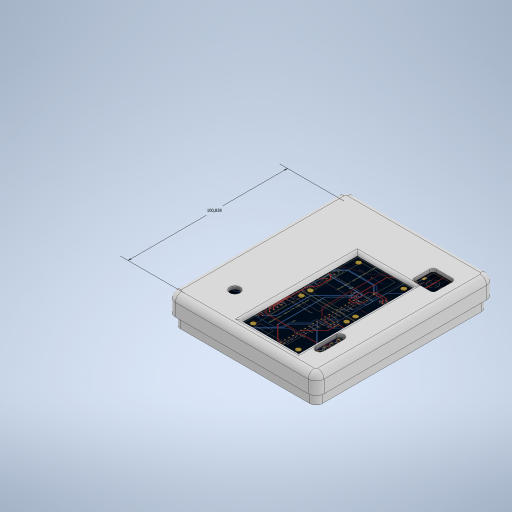
# Autodesk Inventor part: lid_lautering_tank
Saved by Autodesk Inventor 2024.4 (Build 284460000, 460)
## iProperties
Created: 2026-05-24
Part Number: lid_lautering_tank
Material: Generic
Document SubType Name: Modeling
Designer: Emil
Density: 1 g/cm^3
Appearance: Default
Author: Emil
Autodesk Inventor part; units mm, degrees
ref_plane "YZ Plane" through (0, 0, 0) normal (1, 0, 0) x (0, 1, 0)
ref_plane "XZ Plane" through (0, 0, 0) normal (0, 1, 0) x (-1, 0, 0)
ref_plane "XY Plane" through (0, 0, 0) normal (0, 0, 1) x (1, 0, 0)
sketch "Sketch1" plane through (0, 0, 0) normal (0, 1, 0) x (-1, 0, 0)
  line L0 (0, 0) -> (0, -100.838) construction
  line L1 (0, -100.838) -> (-82.0304, -100.838) construction
  line L2 (-82.0304, -100.838) -> (-82.0304, 0) construction
  line L3 (-82.0304, 0) -> (0, 0) construction
  dimension "d3" = 100.838
  constraints: 2 other
  measures "d3" distance of L0.start L0.end
sketch "Sketch2" plane through (0, 0, 0) normal (0, 1, 0) x (-1, 0, 0)
  line L0 (0, 0) -> (0, -100.838) construction
  line L1 (-82.0304, 0) -> (0, 0) construction
  line L2 (0, -100.838) -> (-82.0304, -100.838) construction
  line L3 (-82.0304, -100.838) -> (-82.0304, 0) construction
  line L4 (0, -50.419) -> (-82.0304, -50.419) construction
  line L5 (-41.0152, -50.419) -> (-41.0152, -100.838) construction
  line L6 (-41.0152, -50.419) -> (-41.0152, 0) construction
  line L7 (-85.8804, 3.85) -> (3.85, 3.85)
  line L8 (3.85, 3.85) -> (3.85, -104.688)
  line L9 (3.85, -104.688) -> (-85.8804, -104.688)
  line L10 (-85.8804, -104.688) -> (-85.8804, 3.85)
  line L11 (-85.8804, 3.85) -> (3.85, -104.688) construction
  line L12 (3.85, 3.85) -> (-85.8804, -104.688) construction
  line L13 (-88.0304, 6) -> (6, 6)
  line L14 (6, 6) -> (6, -106.838)
  line L15 (6, -106.838) -> (-88.0304, -106.838)
  line L16 (-88.0304, -106.838) -> (-88.0304, 6)
  line L17 (-88.0304, 6) -> (6, -106.838) construction
  line L18 (6, 6) -> (-88.0304, -106.838) construction
  dimension "d8" = 2.15
  dimension "d9" = 3.85
  dimension "d10" = 3.85
  dimension "d11" = 2.15
  dimension "d39" = 94.0304
  dimension "d40" = 112.838
  constraints: 30 end point, 9 midpoint, 4 parallel, 2 horizontal, 2 perpendicular, 1 other
  measures "d8" distance between parallel lines of L8 L14
  measures "d9" distance between parallel lines of L2 L9
  measures "d10" distance between parallel lines of L8 L0
  measures "d11" distance between parallel lines of L9 L15
  measures "d39" distance of L13.start L13.end
  measures "d40" distance of L15.end L13.start
extrude "Extrusion1" add sketch "Sketch2" against normal blind 10
sketch "Sketch3" plane through (0, 0, 0) normal (0, 1, 0) x (1, 0, 0)
  line L0 (88.0304, -6) -> (-6, -6) projected
  line L1 (-6, 106.838) -> (88.0304, 106.838) projected
  line L2 (-6, -6) -> (88.0304, -6)
  line L3 (88.0304, -6) -> (88.0304, 106.838)
  line L4 (88.0304, 106.838) -> (-6, 106.838)
  line L5 (-6, 106.838) -> (-6, -6)
  point P0 (0, 0)
  point P1 (88.0304, -6)
  point P2 (-6, 106.838)
  constraints: 8 end point, 2 parallel, 1 horizontal, 1 perpendicular
extrude "Extrusion2" add sketch "Sketch3" along normal blind 2
sketch "Sketch4" plane through (0, 0, 0) normal (0, -1, 0) x (1, 0, 0)
  line L0 (69.1573, -1.8666) -> (33.0778, -1.8666)
  line L1 (33.0778, -1.8666) -> (33.0778, -74.9423)
  line L2 (33.0778, -74.9423) -> (69.1573, -74.9423)
  line L3 (69.1573, -74.9423) -> (69.1573, -1.8666)
  line L4 (79.4199, -76.7582) -> (65.2387, -76.7582)
  line L5 (65.2387, -76.7582) -> (65.2387, -90.7941)
  line L6 (65.2387, -90.7941) -> (79.4199, -90.7941)
  line L7 (79.4199, -90.7941) -> (79.4199, -76.7582)
  line L8 (76.6779, -7.6788) -> (71.4655, -7.6788)
  line L9 (71.4655, -7.6788) -> (71.4655, -25.7601)
  line L10 (71.4655, -25.7601) -> (76.6779, -25.7601)
  line L11 (76.6779, -25.7601) -> (76.6779, -7.6788)
  circle A0 centre (15.0393, -15.6107) radius 3.25
  point P0 (0, 0)
  dimension "d34" = 6.5
  constraints: 24 end point, 6 parallel, 3 horizontal, 3 perpendicular, 1 centre point
  measures "d34" diameter of A0
extrude "Extrusion3" cut sketch "Sketch4" against normal blind 2
fillet "Fillet3" radius 4 4 edges at (-6, 2, -50.419) (41.0152, 2, 6) (88.0304, 2, -50.419) (41.0152, 2, -106.838)
fillet "Fillet4" radius 2.6 4 edges at (71.4655, 1, -25.7601) (76.6779, 1, -25.7601) (71.4655, 1, -7.6788) (76.6779, 1, -7.6788)
fillet "Fillet5" radius 2 4 edges at (65.2387, 1, -90.7941) (65.2387, 1, -76.7582) (79.4199, 1, -90.7941) (79.4199, 1, -76.7582)
sketch "Sketch6" plane through (0, -10, 0) normal (0, -1, 0) x (1, 0, 0)
  line L0 (-3.85, -104.688) -> (-3.85, 3.85) projected
  line L1 (-3.85, 3.85) -> (85.8804, 3.85) projected
  line L2 (85.8804, -104.688) -> (-3.85, -104.688) projected
  line L3 (85.8804, 3.85) -> (85.8804, -104.688) projected
  line L4 (85.8804, -104.688) -> (-3.85, -104.688)
  line L5 (-3.85, -104.688) -> (-3.85, 3.85)
  line L6 (-3.85, 3.85) -> (85.8804, 3.85)
  line L7 (85.8804, 3.85) -> (85.8804, -104.688)
  line L8 (84.4315, -102.688) -> (-1.85, -102.688)
  line L9 (-1.85, -102.688) -> (-1.85, 2.5626)
  line L10 (-1.85, 2.5626) -> (84.4315, 2.5626)
  line L11 (84.4315, 2.5626) -> (84.4315, -102.688)
  line L12 (-6, -106.838) -> (88.0304, -106.838) projected
  line L13 (88.0304, -106.838) -> (88.0304, 6) projected
  line L14 (88.0304, 6) -> (-6, 6) projected
  line L15 (-6, 6) -> (-6, -106.838) projected
  line L16 (-3.85, 3.85) -> (85.8804, 3.85) projected
  line L17 (85.8804, 3.85) -> (85.8804, -104.688) projected
  line L18 (85.8804, -104.688) -> (-3.85, -104.688) projected
  line L19 (-3.85, -104.688) -> (-3.85, 3.85)
  point P0 (0, 0)
  point P1 (-4, -101.838)
  point P2 (83.0304, 4)
  point P3 (-1, -104.838)
  point P4 (86.0304, 1)
  dimension "d24" = 2
  dimension "d25" = 2
  constraints: 18 end point, 4 parallel, 2 horizontal, 2 perpendicular, 5 other
extrude "Extrusion4" add sketch "Sketch6" along normal blind 7 and the other way blind 10 contours L0 L1 L3 L2
fillet "Fillet6" radius 4 8 edges at (85.8804, -13.5, 3.85) (84.4315, -8.5, 2.5626) (84.4315, -8.5, -102.688) (85.8804, -13.5, -104.688) (-3.85, -13.5, -104.688) (-1.85, -8.5, -102.688) (-1.85, -8.5, 2.5626) (-3.85, -13.5, 3.85)
fillet "Fillet7" radius 4 8 edges at (41.2908, 0, 2.5626) (-0.6784, 0, 1.391) (-1.85, 0, -50.0627) (-0.6784, 0, -101.5164) (41.2908, 0, -102.688) (83.2599, 0, -101.5164) (84.4315, 0, -50.0627) (83.2599, 0, 1.391)
fillet "Fillet8" radius 2 4 edges at (33.0778, 2, -38.4044) (51.1176, 2, -74.9423) (51.1176, 2, -1.8666) (69.1573, 2, -38.4044)
fillet "Fillet9" radius 5 8 edges at (-4.8284, 0.8284, -105.6664) (-6, -6, -106.838) (-4.8284, 0.8284, 4.8284) (-6, -6, 6) (86.8589, 0.8284, 4.8284) (88.0304, -6, 6) (86.8589, 0.8284, -105.6664) (88.0304, -6, -106.838)
body "Solid1"
